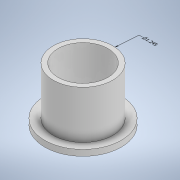
# Autodesk Inventor part: InteriorDustCover
Saved by Autodesk Inventor 2021.2 (Build 252289000, 289)
## iProperties
Created: 2020-02-25
Part Number: InteriorDustCover
Material: Generic
Document SubType Name: Modeling
Designer: robst
Density: 1 g/cm^3
Appearance: Default
Author: robst
Autodesk Inventor part; units mm, degrees
ref_plane "YZ Plane" through (0, 0, 0) normal (1, 0, 0) x (0, 1, 0)
ref_plane "XZ Plane" through (0, 0, 0) normal (0, 1, 0) x (-1, 0, 0)
ref_plane "XY Plane" through (0, 0, 0) normal (0, 0, 1) x (1, 0, 0)
sketch "Sketch1" plane through (0, 0, 0) normal (0, 1, 0) x (-1, 0, 0)
  circle A0 centre (0, 0) radius 20.32
  dimension "d0" = 40.64
  constraints: 1 centre point, 1 coincident
  measures "d0" diameter of A0
extrude "Extrusion1" add sketch "Sketch1" along normal blind 3.175
sketch "Sketch2" plane through (0, 3.175, 0) normal (0, 1, 0) x (1, 0, 0)
  circle A0 centre (0, 0) radius 15.8115
  circle A1 centre (0, 0) radius 13.2715
  dimension "d3" = 31.623
  dimension "d4" = 26.543
  constraints: 2 centre point, 2 coincident
  measures "d3" diameter of A0
  measures "d4" diameter of A1
extrude "Extrusion3" add sketch "Sketch2" along normal blind 25.4
sketch "Sketch3" plane through (0, 3.175, 0) normal (0, 1, 0) x (1, 0, 0)
  circle A0 centre (0, 0) radius 13.2715 construction
  line L0 (-13.2715, 0) -> (13.2715, 0) construction
  line L1 (7.5193, 2.794) -> (10.2454, 2.794)
  line L2 (10.2454, 2.794) -> (10.2454, 2.2234)
  line L3 (10.2454, 2.2234) -> (9.2311, 2.2234)
  line L4 (9.2311, 2.2234) -> (9.2311, -1.5215)
  line L5 (9.2311, -1.5215) -> (10.2454, -1.5215)
  line L6 (10.2454, -1.5215) -> (10.2454, -2.0332)
  spline S0 degree 2 poles (10.2454, -2.0332) (9.6703, -2.0332) (9.1269, -2.3593) (9.0907, -2.8121) knots 0 0 0 1 2 2 2
  line L7 (9.0907, -2.8121) -> (8.5111, -2.8121)
  line L8 (8.5111, -2.8121) -> (8.5111, 2.2234)
  line L9 (8.5111, 2.2234) -> (7.5193, 2.2234)
  line L10 (7.5193, 2.2234) -> (7.5193, 2.794)
  line L11 (5.2914, 2.794) -> (6.188, 2.794)
  line L12 (6.188, 2.794) -> (6.188, 1.7253)
  line L13 (6.188, 1.7253) -> (5.2914, 1.7253)
  line L14 (5.2914, 1.7253) -> (5.2914, 2.794)
  line L15 (0.7177, 2.794) -> (4.1638, 2.794)
  line L16 (4.1638, 2.794) -> (4.1638, 2.0015)
  spline S1 degree 2 poles (4.1638, 2.0015) (3.7925, 1.6529) (3.1314, 1.0053) (2.8144, 0.6566) knots 0 0 0 1 2 2 2
  spline S2 degree 2 poles (2.8144, 0.6566) (2.1759, -0.0453) (1.7095, -0.8876) (1.7095, -1.3359) knots 0 0 0 1 2 2 2
  spline S3 degree 2 poles (1.7095, -1.3359) (1.7095, -1.5713) (1.8544, -1.9246) (1.9857, -2.0378) knots 0 0 0 1 2 2 2
  spline S4 degree 2 poles (1.9857, -2.0378) (2.117, -2.151) (2.4612, -2.2642) (2.6695, -2.2642) knots 0 0 0 1 2 2 2
  spline S5 degree 2 poles (2.6695, -2.2642) (2.8687, -2.2642) (3.2763, -2.1646) (3.4619, -2.0876) knots 0 0 0 1 2 2 2
  spline S6 degree 2 poles (3.4619, -2.0876) (3.6204, -2.0242) (3.9148, -1.843) (4.0053, -1.7796) knots 0 0 0 1 2 2 2
  line L17 (4.0053, -1.7796) -> (4.0461, -1.7796)
  line L18 (4.0461, -1.7796) -> (4.0461, -2.5766)
  spline S7 degree 2 poles (4.0461, -2.5766) (3.8151, -2.6898) (2.9865, -2.9117) (2.6151, -2.9117) knots 0 0 0 1 2 2 2
  spline S8 degree 2 poles (2.6151, -2.9117) (1.8317, -2.9117) (0.9487, -2.083) (0.9487, -1.3766) knots 0 0 0 1 2 2 2
  spline S9 degree 2 poles (0.9487, -1.3766) (0.9487, -1.0461) (1.1027, -0.4936) (1.2385, -0.2581) knots 0 0 0 1 2 2 2
  spline S10 degree 2 poles (1.2385, -0.2581) (1.3744, -0.0136) (1.7683, 0.4664) (1.9857, 0.6974) knots 0 0 0 1 2 2 2
  spline S11 degree 2 poles (1.9857, 0.6974) (2.3389, 1.0823) (3.2038, 1.9064) (3.4619, 2.1464) knots 0 0 0 1 2 2 2
  line L19 (3.4619, 2.1464) -> (0.7177, 2.1464)
  line L20 (0.7177, 2.1464) -> (0.7177, 2.794)
  line L21 (-3.625, 0.874) -> (-2.9593, 0.874)
  line L22 (-2.9593, 0.874) -> (-2.9593, 2.794)
  line L23 (-2.9593, 2.794) -> (-2.2393, 2.794)
  line L24 (-2.2393, 2.794) -> (-2.2393, 0.874)
  line L25 (-2.2393, 0.874) -> (0.2287, 0.874)
  line L26 (0.2287, 0.874) -> (0.2287, 0.086)
  line L27 (0.2287, 0.086) -> (-2.271, -2.794)
  line L28 (-2.271, -2.794) -> (-2.9593, -2.794)
  line L29 (-2.9593, -2.794) -> (-2.9593, 0.2717)
  line L30 (-2.9593, 0.2717) -> (-3.625, 0.2717)
  line L31 (-3.625, 0.2717) -> (-3.625, 0.874)
  line L32 (-2.2393, 0.2717) -> (-2.2393, -1.911)
  line L33 (-2.2393, -1.911) -> (-0.36, 0.2717)
  line L34 (-0.36, 0.2717) -> (-2.2393, 0.2717)
  spline S12 degree 2 poles (-7.6099, 1.0189) (-7.6099, 1.4219) (-7.3518, 2.1102) (-7.1163, 2.3638) knots 0 0 0 1 2 2 2
  spline S13 degree 2 poles (-7.1163, 2.3638) (-6.8808, 2.6174) (-6.179, 2.9117) (-5.7442, 2.9117) knots 0 0 0 1 2 2 2
  spline S14 degree 2 poles (-5.7442, 2.9117) (-5.3457, 2.9117) (-4.5669, 2.7351) (-4.2816, 2.5948) knots 0 0 0 1 2 2 2
  line L35 (-4.2816, 2.5948) -> (-4.2816, 1.8023)
  line L36 (-4.2816, 1.8023) -> (-4.3359, 1.8023)
  spline S15 degree 2 poles (-4.3359, 1.8023) (-4.4219, 1.8657) (-4.7435, 2.0287) (-4.9382, 2.1012) knots 0 0 0 1 2 2 2
  spline S16 degree 2 poles (-4.9382, 2.1012) (-5.1601, 2.1781) (-5.5269, 2.2642) (-5.7578, 2.2642) knots 0 0 0 1 2 2 2
  spline S17 degree 2 poles (-5.7578, 2.2642) (-5.9842, 2.2642) (-6.4099, 2.1012) (-6.5639, 1.9246) knots 0 0 0 1 2 2 2
  spline S18 degree 2 poles (-6.5639, 1.9246) (-6.7042, 1.757) (-6.8491, 1.3132) (-6.8491, 1.0144) knots 0 0 0 1 2 2 2
  spline S19 degree 2 poles (-6.8491, 1.0144) (-6.8491, 0.7155) (-6.6861, 0.3351) (-6.5322, 0.2083) knots 0 0 0 1 2 2 2
  spline S20 degree 2 poles (-6.5322, 0.2083) (-6.3737, 0.0679) (-5.9027, -0.0498) (-5.6174, -0.0498) knots 0 0 0 1 2 2 2
  spline S21 degree 2 poles (-5.6174, -0.0498) (-5.3095, -0.0498) (-4.6982, 0.0453) (-4.5125, 0.086) knots 0 0 0 1 2 2 2
  line L37 (-4.5125, 0.086) -> (-4.5125, -2.794)
  line L38 (-4.5125, -2.794) -> (-7.5782, -2.794)
  line L39 (-7.5782, -2.794) -> (-7.5782, -2.1374)
  line L40 (-7.5782, -2.1374) -> (-5.2325, -2.1374)
  line L41 (-5.2325, -2.1374) -> (-5.2325, -0.6476)
  spline S22 degree 2 poles (-5.2325, -0.6476) (-5.3684, -0.6657) (-5.631, -0.6793) (-5.7397, -0.6793) knots 0 0 0 1 2 2 2
  spline S23 degree 2 poles (-5.7397, -0.6793) (-6.1699, -0.6793) (-6.7631, -0.5389) (-7.0348, -0.3306) knots 0 0 0 1 2 2 2
  spline S24 degree 2 poles (-7.0348, -0.3306) (-7.311, -0.1223) (-7.6099, 0.5117) (-7.6099, 1.0189) knots 0 0 0 1 2 2 2
  line L42 (-9.2537, -3.0431) -> (-9.0907, -0.8694)
  line L43 (-9.0907, -0.8694) -> (-8.5971, -0.8694)
  line L44 (-8.5971, -0.8694) -> (-8.4341, -3.0431)
  line L45 (-8.4341, -3.0431) -> (-9.2537, -3.0431)
  line L46 (-10.6666, -3.0431) -> (-10.5035, -0.8694)
  line L47 (-10.5035, -0.8694) -> (-10.0099, -0.8694)
  line L48 (-10.0099, -0.8694) -> (-9.8469, -3.0431)
  line L49 (-9.8469, -3.0431) -> (-10.6666, -3.0431)
  constraints: 2 end point, 2 horizontal, 2 point on circle
extrude "Extrusion4" add sketch "Sketch3" along normal blind 0.635
sketch "Sketch4" plane through (0, 0, 0) normal (0, -1, 0) x (1, 0, 0)
  circle A0 centre (0, 0) radius 20.32 construction
  line L0 (20.32, 0) -> (-20.32, 0) construction
  spline S0 degree 2 poles (-11.2447, -3.9459) (-12.0722, -3.9459) (-13.2331, -3.6) (-13.7456, -3.353) knots 0 0 0 1 2 2 2
  line L1 (-13.7456, -3.353) -> (-13.7456, -2.081)
  line L2 (-13.7456, -2.081) -> (-13.6715, -2.081)
  spline S1 degree 2 poles (-13.6715, -2.081) (-13.1714, -2.5503) (-11.9055, -3.069) (-11.3188, -3.069) knots 0 0 0 1 2 2 2
  spline S2 degree 2 poles (-11.3188, -3.069) (-10.479, -3.069) (-9.6207, -2.3712) (-9.6207, -1.7969) knots 0 0 0 1 2 2 2
  spline S3 degree 2 poles (-9.6207, -1.7969) (-9.6207, -1.34) (-10.0715, -0.7719) (-10.5593, -0.6299) knots 0 0 0 1 2 2 2
  spline S4 degree 2 poles (-10.5593, -0.6299) (-10.9113, -0.5311) (-11.4979, -0.3952) (-11.9364, -0.2841) knots 0 0 0 1 2 2 2
  spline S5 degree 2 poles (-11.9364, -0.2841) (-12.3316, -0.1791) (-12.9552, 0.1359) (-13.1961, 0.389) knots 0 0 0 1 2 2 2
  spline S6 degree 2 poles (-13.1961, 0.389) (-13.4307, 0.6422) (-13.6901, 1.3215) (-13.6901, 1.7661) knots 0 0 0 1 2 2 2
  spline S7 degree 2 poles (-13.6901, 1.7661) (-13.6901, 2.6923) (-12.2451, 3.9459) (-11.1274, 3.9459) knots 0 0 0 1 2 2 2
  spline S8 degree 2 poles (-11.1274, 3.9459) (-10.4852, 3.9459) (-9.349, 3.6927) (-8.8612, 3.4518) knots 0 0 0 1 2 2 2
  line L3 (-8.8612, 3.4518) -> (-8.8612, 2.2415)
  line L4 (-8.8612, 2.2415) -> (-8.9353, 2.2415)
  spline S9 degree 2 poles (-8.9353, 2.2415) (-9.2996, 2.575) (-10.4358, 3.069) (-11.0595, 3.069) knots 0 0 0 1 2 2 2
  spline S10 degree 2 poles (-11.0595, 3.069) (-11.7635, 3.069) (-12.6341, 2.4083) (-12.6341, 1.871) knots 0 0 0 1 2 2 2
  spline S11 degree 2 poles (-12.6341, 1.871) (-12.6341, 1.3894) (-12.1216, 0.8151) (-11.64, 0.6854) knots 0 0 0 1 2 2 2
  spline S12 degree 2 poles (-11.64, 0.6854) (-11.3188, 0.599) (-10.3864, 0.3767) (-10.0777, 0.2841) knots 0 0 0 1 2 2 2
  spline S13 degree 2 poles (-10.0777, 0.2841) (-9.2934, 0.0432) (-8.5648, -0.9263) (-8.5648, -1.6364) knots 0 0 0 1 2 2 2
  spline S14 degree 2 poles (-8.5648, -1.6364) (-8.5648, -2.0872) (-8.9291, -2.9517) (-9.2564, -3.2542) knots 0 0 0 1 2 2 2
  spline S15 degree 2 poles (-9.2564, -3.2542) (-9.6207, -3.5877) (-10.547, -3.9459) (-11.2447, -3.9459) knots 0 0 0 1 2 2 2
  spline S16 degree 2 poles (-5.8786, -3.9212) (-6.6629, -3.9212) (-7.5459, -3.0258) (-7.5459, -2.0563) knots 0 0 0 1 2 2 2
  line L5 (-7.5459, -2.0563) -> (-7.5459, 1.1115)
  line L6 (-7.5459, 1.1115) -> (-8.1943, 1.1115)
  line L7 (-8.1943, 1.1115) -> (-8.1943, 1.9081)
  line L8 (-8.1943, 1.9081) -> (-7.5459, 1.9081)
  line L9 (-7.5459, 1.9081) -> (-7.5459, 3.5506)
  line L10 (-7.5459, 3.5506) -> (-6.5826, 3.5506)
  line L11 (-6.5826, 3.5506) -> (-6.5826, 1.9081)
  line L12 (-6.5826, 1.9081) -> (-4.8104, 1.9081)
  line L13 (-4.8104, 1.9081) -> (-4.8104, 1.1115)
  line L14 (-4.8104, 1.1115) -> (-6.5826, 1.1115)
  line L15 (-6.5826, 1.1115) -> (-6.5826, -1.6117)
  spline S17 degree 2 poles (-6.5826, -1.6117) (-6.5826, -2.0439) (-6.5517, -2.5194) (-6.4467, -2.7232) knots 0 0 0 1 2 2 2
  spline S18 degree 2 poles (-6.4467, -2.7232) (-6.3603, -2.9023) (-5.9713, -3.0813) (-5.6378, -3.0813) knots 0 0 0 1 2 2 2
  spline S19 degree 2 poles (-5.6378, -3.0813) (-5.4032, -3.0813) (-4.9647, -2.9393) (-4.8659, -2.8961) knots 0 0 0 1 2 2 2
  line L16 (-4.8659, -2.8961) -> (-4.8104, -2.8961)
  line L17 (-4.8104, -2.8961) -> (-4.8104, -3.7606)
  spline S20 degree 2 poles (-4.8104, -3.7606) (-5.0821, -3.8347) (-5.6378, -3.9212) (-5.8786, -3.9212) knots 0 0 0 1 2 2 2
  spline S21 degree 2 poles (-1.6179, -3.9397) (-2.9887, -3.9397) (-4.4954, -2.4021) (-4.4954, -0.9818) knots 0 0 0 1 2 2 2
  spline S22 degree 2 poles (-4.4954, -0.9818) (-4.4954, 0.4137) (-3.0319, 2.0686) (-1.8525, 2.0686) knots 0 0 0 1 2 2 2
  spline S23 degree 2 poles (-1.8525, 2.0686) (-1.3215, 2.0686) (-0.5002, 1.7599) (-0.1976, 1.4326) knots 0 0 0 1 2 2 2
  spline S24 degree 2 poles (-0.1976, 1.4326) (0.1112, 1.1053) (0.4384, 0.1606) (0.4384, -0.5249) knots 0 0 0 1 2 2 2
  line L18 (0.4384, -0.5249) -> (0.4384, -1.0498)
  line L19 (0.4384, -1.0498) -> (-3.5198, -1.0498)
  spline S25 degree 2 poles (-3.5198, -1.0498) (-3.5198, -2.0439) (-2.5194, -3.0999) (-1.6302, -3.0999) knots 0 0 0 1 2 2 2
  spline S26 degree 2 poles (-1.6302, -3.0999) (-1.3153, -3.0999) (-0.704, -2.9578) (-0.457, -2.8467) knots 0 0 0 1 2 2 2
  spline S27 degree 2 poles (-0.457, -2.8467) (-0.1976, -2.7232) (0.1606, -2.5071) (0.2779, -2.4083) knots 0 0 0 1 2 2 2
  line L20 (0.2779, -2.4083) -> (0.3335, -2.4083)
  line L21 (0.3335, -2.4083) -> (0.3335, -3.458)
  spline S28 degree 2 poles (0.3335, -3.458) (0.1667, -3.5259) (-0.3396, -3.7235) (-0.5372, -3.7791) knots 0 0 0 1 2 2 2
  spline S29 degree 2 poles (-0.5372, -3.7791) (-0.8151, -3.8594) (-1.2721, -3.9397) (-1.6179, -3.9397) knots 0 0 0 1 2 2 2
  spline S30 degree 2 poles (-0.5002, -0.3149) (-0.5125, 0.0741) (-0.6731, 0.6422) (-0.8275, 0.8336) knots 0 0 0 1 2 2 2
  spline S31 degree 2 poles (-0.8275, 0.8336) (-0.9942, 1.0498) (-1.5191, 1.2782) (-1.9081, 1.2782) knots 0 0 0 1 2 2 2
  spline S32 degree 2 poles (-1.9081, 1.2782) (-2.2909, 1.2782) (-2.8282, 1.0498) (-3.0505, 0.8275) knots 0 0 0 1 2 2 2
  spline S33 degree 2 poles (-3.0505, 0.8275) (-3.2666, 0.599) (-3.4889, 0.0494) (-3.5198, -0.3149) knots 0 0 0 1 2 2 2
  line L22 (-3.5198, -0.3149) -> (-0.5002, -0.3149)
  spline S34 degree 2 poles (3.8965, -3.9397) (2.5256, -3.9397) (1.0189, -2.4021) (1.0189, -0.9818) knots 0 0 0 1 2 2 2
  spline S35 degree 2 poles (1.0189, -0.9818) (1.0189, 0.4137) (2.4824, 2.0686) (3.6618, 2.0686) knots 0 0 0 1 2 2 2
  spline S36 degree 2 poles (3.6618, 2.0686) (4.1929, 2.0686) (5.0141, 1.7599) (5.3167, 1.4326) knots 0 0 0 1 2 2 2
  spline S37 degree 2 poles (5.3167, 1.4326) (5.6255, 1.1053) (5.9527, 0.1606) (5.9527, -0.5249) knots 0 0 0 1 2 2 2
  line L23 (5.9527, -0.5249) -> (5.9527, -1.0498)
  line L24 (5.9527, -1.0498) -> (1.9945, -1.0498)
  spline S38 degree 2 poles (1.9945, -1.0498) (1.9945, -2.0439) (2.9949, -3.0999) (3.8841, -3.0999) knots 0 0 0 1 2 2 2
  spline S39 degree 2 poles (3.8841, -3.0999) (4.199, -3.0999) (4.8104, -2.9578) (5.0574, -2.8467) knots 0 0 0 1 2 2 2
  spline S40 degree 2 poles (5.0574, -2.8467) (5.3167, -2.7232) (5.6749, -2.5071) (5.7922, -2.4083) knots 0 0 0 1 2 2 2
  line L25 (5.7922, -2.4083) -> (5.8478, -2.4083)
  line L26 (5.8478, -2.4083) -> (5.8478, -3.458)
  spline S41 degree 2 poles (5.8478, -3.458) (5.681, -3.5259) (5.1747, -3.7235) (4.9771, -3.7791) knots 0 0 0 1 2 2 2
  spline S42 degree 2 poles (4.9771, -3.7791) (4.6992, -3.8594) (4.2423, -3.9397) (3.8965, -3.9397) knots 0 0 0 1 2 2 2
  spline S43 degree 2 poles (5.0141, -0.3149) (5.0018, 0.0741) (4.8412, 0.6422) (4.6869, 0.8336) knots 0 0 0 1 2 2 2
  spline S44 degree 2 poles (4.6869, 0.8336) (4.5201, 1.0498) (3.9953, 1.2782) (3.6062, 1.2782) knots 0 0 0 1 2 2 2
  spline S45 degree 2 poles (3.6062, 1.2782) (3.2234, 1.2782) (2.6861, 1.0498) (2.4638, 0.8275) knots 0 0 0 1 2 2 2
  spline S46 degree 2 poles (2.4638, 0.8275) (2.2477, 0.599) (2.0254, 0.0494) (1.9945, -0.3149) knots 0 0 0 1 2 2 2
  line L27 (1.9945, -0.3149) -> (5.0141, -0.3149)
  line L28 (7.9102, -3.81) -> (6.9469, -3.81)
  line L29 (6.9469, -3.81) -> (6.9469, 4.1496)
  line L30 (6.9469, 4.1496) -> (7.9102, 4.1496)
  line L31 (7.9102, 4.1496) -> (7.9102, -3.81)
  spline S47 degree 2 poles (11.8067, -3.9397) (10.4358, -3.9397) (8.9291, -2.4021) (8.9291, -0.9818) knots 0 0 0 1 2 2 2
  spline S48 degree 2 poles (8.9291, -0.9818) (8.9291, 0.4137) (10.3926, 2.0686) (11.572, 2.0686) knots 0 0 0 1 2 2 2
  spline S49 degree 2 poles (11.572, 2.0686) (12.1031, 2.0686) (12.9244, 1.7599) (13.2269, 1.4326) knots 0 0 0 1 2 2 2
  spline S50 degree 2 poles (13.2269, 1.4326) (13.5357, 1.1053) (13.863, 0.1606) (13.863, -0.5249) knots 0 0 0 1 2 2 2
  line L32 (13.863, -0.5249) -> (13.863, -1.0498)
  line L33 (13.863, -1.0498) -> (9.9048, -1.0498)
  spline S51 degree 2 poles (9.9048, -1.0498) (9.9048, -2.0439) (10.9051, -3.0999) (11.7943, -3.0999) knots 0 0 0 1 2 2 2
  spline S52 degree 2 poles (11.7943, -3.0999) (12.1093, -3.0999) (12.7206, -2.9578) (12.9676, -2.8467) knots 0 0 0 1 2 2 2
  spline S53 degree 2 poles (12.9676, -2.8467) (13.2269, -2.7232) (13.5851, -2.5071) (13.7024, -2.4083) knots 0 0 0 1 2 2 2
  line L34 (13.7024, -2.4083) -> (13.758, -2.4083)
  line L35 (13.758, -2.4083) -> (13.758, -3.458)
  spline S54 degree 2 poles (13.758, -3.458) (13.5913, -3.5259) (13.0849, -3.7235) (12.8873, -3.7791) knots 0 0 0 1 2 2 2
  spline S55 degree 2 poles (12.8873, -3.7791) (12.6094, -3.8594) (12.1525, -3.9397) (11.8067, -3.9397) knots 0 0 0 1 2 2 2
  spline S56 degree 2 poles (12.9244, -0.3149) (12.912, 0.0741) (12.7515, 0.6422) (12.5971, 0.8336) knots 0 0 0 1 2 2 2
  spline S57 degree 2 poles (12.5971, 0.8336) (12.4304, 1.0498) (11.9055, 1.2782) (11.5165, 1.2782) knots 0 0 0 1 2 2 2
  spline S58 degree 2 poles (11.5165, 1.2782) (11.1336, 1.2782) (10.5964, 1.0498) (10.3741, 0.8275) knots 0 0 0 1 2 2 2
  spline S59 degree 2 poles (10.3741, 0.8275) (10.1579, 0.599) (9.9356, 0.0494) (9.9048, -0.3149) knots 0 0 0 1 2 2 2
  line L36 (9.9048, -0.3149) -> (12.9244, -0.3149)
  constraints: 2 end point, 2 horizontal, 2 point on circle
extrude "Extrusion5" cut sketch "Sketch4" against normal blind 1.27
equation "\"d0\" = outerDiameter"
equation "\"d1\" = supportThickness"
equation "\"d3\" = eyepieceOuterDiameter"
equation "\"d4\" = eyepieceInnerDiameter"
equation "\"d7\" = insertHeight"
equation "\"d11\" = textHeight"
equation "\"d17\" = textDepth"
equation "\"eyepieceOuterDiameter\" = 31.623"
equation "\"wallThickness\" = 2.54"
equation "\"eyepieceInnerDiameter\" = eyepieceOuterDiameter - 2 * wallThickness"
equation "\"outerDiameter\" = 40.64"
equation "\"supportThickness\" = 3.175"
equation "\"insertHeight\" = 25.4"
equation "\"textDepth\" = 1.27"
equation "\"textHeight\" = 0.635"
body "Solid1"
